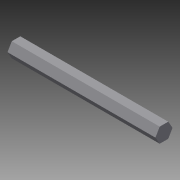
# Autodesk Inventor part: axle
Saved by Autodesk Inventor 2015 SP1 (Build 190203100, 203)
## iProperties
Created: 2014-12-22
Part Number: axle
Material: Generic
Document SubType Name: Modeling
Designer: Jarod
Density: 1 g/cm^3
Appearance: Default
Author: Jarod
Autodesk Inventor part; units mm, degrees
ref_plane "YZ Plane" through (0, 0, 0) normal (1, 0, 0) x (0, 1, 0)
ref_plane "XZ Plane" through (0, 0, 0) normal (0, 1, 0) x (-1, 0, 0)
ref_plane "XY Plane" through (0, 0, 0) normal (0, 0, 1) x (1, 0, 0)
sketch "Sketch1" plane through (0, 0, 0) normal (1, 0, 0) x (0, 1, 0)
  circle A0 centre (0, 0) radius 6.35 construction
  line L0 (0, 0) -> (6.35, -3.6662) construction
  line L1 (0, 0) -> (7.3323, 0) construction
  line L2 (0, 0) -> (6.35, 3.6662) construction
  line L3 (0, 0) -> (7.3323, 0) construction
  line L4 (0, 0) -> (6.35, 3.6662) construction
  line L5 (0, 0) -> (0, 7.3323) construction
  line L6 (0, 0) -> (-6.35, 3.6662) construction
  line L7 (0, 0) -> (-6.35, -3.6662) construction
  line L8 (0, 0) -> (0, -7.3323) construction
  line L9 (0, 7.3323) -> (6.35, 3.6662)
  line L10 (6.35, 3.6662) -> (6.35, -3.6662)
  line L11 (6.35, -3.6662) -> (0, -7.3323)
  line L12 (0, -7.3323) -> (-6.35, -3.6662)
  line L13 (-6.35, -3.6662) -> (-6.35, 3.6662)
  line L14 (-6.35, 3.6662) -> (0, 7.3323)
  dimension "d0" = 12.7
  dimension "d1" = 30
  dimension "d2" = 30
  dimension "d5" = 360
  constraints: 30 end point, 3 parallel, 2 equal length, 2 horizontal, 1 centre point, 1 coincident, 19 other
  measures "d0" diameter of A0
  measures "d1" angle of L0 L1
  measures "d2" angle of L3 L2
extrude "Extrusion1" add sketch "Sketch1" along normal blind 152.4
body "Solid1"
